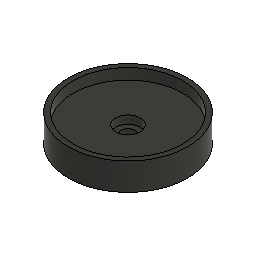
foot (Autodesk Fusion 360 design; units mm, degrees)
Autodesk Fusion 360 part; units mm, degrees
sketch "Skizze1" plane through (0, 0, 0) normal (0, 0, 1) x (1, 0, 0)
  line L0 (-39.8802, 0) -> (43.6662, 0) construction
  line L1 (0, 41.7732) -> (0, -47.5785) construction
  circle A0 centre (0, 0) radius 11
  circle A1 centre (0, 0) radius 10.1
  circle A2 centre (0, 0) radius 1.25
  circle A3 centre (0, 0) radius 2.25
  dimension "d1" = 22
  dimension "d2" = 20.2
  dimension "d3" = 2.5
  dimension "d4" = 4.5
  constraint horizontal L0
  constraint perpendicular L0 L1
  constraint coincident A0.centre L0
  constraint coincident A0.centre L1
  constraint coincident A0.centre A1.centre
  measures "d1" diameter of A0
  measures "d2" diameter of A1
  measures "d3" diameter of A2
  measures "d4" diameter of A3
extrude "Extrusion1" add sketch "Skizze1" against normal blind 1.5 contours A1 | A3
extrude "Extrusion2" add sketch "Skizze1" along normal blind 1.5 contours A1
extrude "Extrusion3" add sketch "Skizze1" along normal blind 3.5 and the other way blind 1.5 contours A0
named bodies: "foot"
